五金工具收纳_镂空1 (Autodesk Fusion 360 design; units mm, degrees)
part number: 2026-02-27-19-53-02-708
Autodesk Fusion 360 part; units mm, degrees
(part 1 of 9)
sketch "草图1" plane through (0, 0, 0) normal (0, 0, 1) x (1, 0, 0)
  line L0 (-120, 120) -> (120, 120)
  line L1 (120, 120) -> (120, -120)
  line L2 (120, -120) -> (-120, -120)
  line L3 (-120, -120) -> (-120, 120)
  line L4 (-120, 120) -> (120, -120) construction
  line L5 (120, 120) -> (-120, -120) construction
  line L6 (-116, -116) -> (-116, 116)
  line L7 (-116, 116) -> (116, 116)
  line L8 (116, 116) -> (116, -116)
  line L9 (116, -116) -> (-116, -116)
  line L10 (-116, 116) -> (4, 116)
  line L11 (4, 116) -> (4, -4)
  line L12 (4, -4) -> (-116, -4)
  line L13 (-116, -4) -> (-116, 116)
  line L14 (7, 116) -> (7, -7)
  line L15 (7, -7) -> (-116, -7)
  line L16 (-91.3834, 29.143) -> (-25.513, 29.143) construction
  line L17 (-25.513, 29.143) -> (-25.513, 88.3753) construction
  line L18 (-25.513, 88.3753) -> (-91.3834, 88.3753) construction
  line L19 (-91.3834, 88.3753) -> (-91.3834, 29.143) construction
  line L20 (7, 80) -> (72, 80)
  line L21 (72, 80) -> (72, 116)
  line L22 (7, 83) -> (69, 83)
  line L23 (69, 83) -> (69, 116)
  line L24 (25.1429, 88.9882) -> (53.1683, 88.9882) construction
  line L25 (53.1683, 88.9882) -> (53.1683, 99.6185) construction
  line L26 (53.1683, 99.6185) -> (25.1429, 99.6185) construction
  line L27 (25.1429, 99.6185) -> (25.1429, 88.9882) construction
  line L28 (67, 80) -> (67, 57)
  line L29 (67, 57) -> (7, 57)
  line L30 (17, 80) -> (57, 80)
  line L31 (57, 80) -> (57, 60)
  line L32 (57, 60) -> (17, 60)
  line L33 (17, 60) -> (17, 80)
  line L34 (26, 65.6005) -> (48.0911, 65.6005) construction
  line L35 (48.0911, 65.6005) -> (48.0911, 73) construction
  line L36 (48.0911, 73) -> (26, 73) construction
  line L37 (26, 73) -> (26, 65.6005) construction
  line L38 (-116, -7) -> (-41, -7)
  line L39 (-41, -7) -> (-41, -82)
  line L40 (-41, -82) -> (-116, -82)
  line L41 (-116, -82) -> (-116, -7)
  line L42 (-38, -7) -> (-38, -85)
  line L43 (-38, -85) -> (-116, -85)
  line L44 (-99.1433, -54.3081) -> (-63.0106, -54.3081) construction
  line L45 (-63.0106, -54.3081) -> (-63.0106, -32.999) construction
  line L46 (-63.0106, -32.999) -> (-99.1433, -32.999) construction
  line L47 (-99.1433, -32.999) -> (-99.1433, -54.3081) construction
  line L48 (7, 57) -> (67, 57)
  line L49 (67, 57) -> (67, 37)
  line L50 (67, 37) -> (7, 37)
  line L51 (7, 37) -> (7, 57)
  line L52 (64, 57) -> (64, 40)
  line L53 (64, 40) -> (7, 40)
  line L54 (25.5114, 42.6447) -> (56.3611, 42.6447) construction
  line L55 (56.3611, 42.6447) -> (56.3611, 51.3132) construction
  line L56 (56.3611, 51.3132) -> (25.5114, 51.3132) construction
  line L57 (25.5114, 51.3132) -> (25.5114, 42.6447) construction
  line L58 (72, 103) -> (116, 103)
  line L59 (72, 87) -> (116, 87)
  line L60 (72, 100) -> (116, 100)
  line L61 (72, 84) -> (116, 84)
  line L62 (67, 71) -> (116, 71)
  line L63 (67, 40) -> (116, 40)
  line L64 (67, 68) -> (116, 68)
  line L65 (67, 37) -> (116, 37)
  line L66 (76.846, 102.1326) -> (102.0197, 102.0197) construction
  line L67 (102.0197, 102.0197) -> (102.0756, 114.498) construction
  line L68 (102.0756, 114.498) -> (76.902, 114.6109) construction
  line L69 (76.902, 114.6109) -> (76.846, 102.1326) construction
  line L70 (84.3585, 90.542) -> (111.7961, 90.6188) construction
  line L71 (111.7961, 90.6188) -> (111.7764, 97.6581) construction
  line L72 (111.7764, 97.6581) -> (84.3388, 97.5814) construction
  line L73 (84.3388, 97.5814) -> (84.3585, 90.542) construction
  line L74 (94.1738, 75) -> (110, 75) construction
  line L75 (110, 75) -> (110, 79.4268) construction
  line L76 (110, 79.4268) -> (94.1738, 79.4268) construction
  line L77 (94.1738, 79.4268) -> (94.1738, 75) construction
  line L78 (80, 47.31) -> (108.2637, 47.31) construction
  line L79 (108.2637, 47.31) -> (108.2637, 60) construction
  line L80 (108.2637, 60) -> (80, 60) construction
  line L81 (80, 60) -> (80, 47.31) construction
  line L82 (-85, -85) -> (-85, -116)
  line L83 (-54, -85) -> (-54, -116)
  line L84 (-38, -85) -> (-5, -85)
  line L85 (-5, -85) -> (-5, -116)
  line L86 (-23, -85) -> (-23, -116)
  line L87 (-116, -85) -> (-85, -116) construction
  line L88 (-54, -85) -> (-85, -116) construction
  line L89 (-85, -85) -> (-54, -116) construction
  line L90 (-54, -85) -> (-23, -116) construction
  line L91 (-23, -116) -> (-5, -85) construction
  line L92 (-23, -85) -> (-5, -116) construction
  line L93 (-23, -85) -> (-54, -116) construction
  circle A0 centre (-100.5, -100.5) radius 3.65
  circle A1 centre (-69.5, -100.5) radius 3.65
  circle A2 centre (-38.5, -100.5) radius 2.25
  circle A3 centre (-14, -100.5) radius 2.5
  line L94 (72, 6) -> (7, 6)
  line L95 (72, 12) -> (72, 6)
  line L96 (26.8319, 6.972) -> (48.9756, 6.972) construction
  line L97 (48.9756, 6.972) -> (48.9756, 11.0156) construction
  line L98 (48.9756, 11.0156) -> (26.8319, 11.0156) construction
  line L99 (26.8319, 11.0156) -> (26.8319, 6.972) construction
  line L100 (40.1808, 17.1326) -> (43.385, 17.1326) construction
  line L101 (43.385, 17.1326) -> (43.385, 35.2897) construction
  line L102 (43.385, 35.2897) -> (40.1808, 35.2897) construction
  line L103 (40.1808, 35.2897) -> (40.1808, 17.1326) construction
  line L104 (18.6537, 18.964) -> (25.5317, 18.964) construction
  line L105 (25.5317, 18.964) -> (25.5317, 32.3581) construction
  line L106 (25.5317, 32.3581) -> (18.6537, 32.3581) construction
  line L107 (18.6537, 32.3581) -> (18.6537, 18.964) construction
  line L108 (35, 37) -> (35, 12)
  line L109 (35, 12) -> (7, 12)
  line L110 (32, 15) -> (7, 15)
  line L111 (32, 37) -> (32, 15)
  line L112 (35, 15) -> (67, 15)
  line L113 (67, 15) -> (67, 37)
  line L114 (35, 12) -> (70, 12)
  line L115 (70, 12) -> (70, 37)
  line L116 (70, 30) -> (116, 30)
  line L117 (70, 27) -> (116, 27)
  line L118 (79.0707, 32.0224) -> (93.9955, 32.0224) construction
  line L119 (93.9955, 32.0224) -> (93.9955, 35.3609) construction
  line L120 (93.9955, 35.3609) -> (79.0707, 35.3609) construction
  line L121 (79.0707, 35.3609) -> (79.0707, 32.0224) construction
  line L122 (7, -7) -> (116, -7)
  line L123 (116, -7) -> (116, -116)
  line L124 (116, -116) -> (7, -116)
  line L125 (7, -116) -> (7, -7)
  line L126 (7, 116) -> (7, 120)
  line L127 (-116, -7) -> (-121.1752, -7)
  line L128 (72, 116) -> (72, 120)
  line L129 (116, 100) -> (120, 100)
  line L130 (116, 84) -> (120, 84)
  line L131 (69, 116) -> (69, 120)
  line L132 (72, 100) -> (69, 100)
  line L133 (72, 84) -> (69, 84)
  line L134 (-38, -7) -> (-38, -4)
  line L135 (-116, -85) -> (-120, -85)
  line L136 (-116, -4) -> (-120, -4)
  line L137 (86.5, 23) -> (86.5, -4)
  line L138 (74.7536, 23) -> (74.7536, 3)
  line L139 (84, -4.0797) -> (84, 23)
  line L140 (113.5, -4) -> (113.5, 23)
  line L141 (86.5, -4) -> (113.5, -4)
  line L142 (113.5, 23) -> (86.5, 23)
  line L143 (84, 23) -> (74.7536, 23)
  line L144 (7, -4.0797) -> (84, -4.0797)
  line L145 (74.7536, 3) -> (7, 3)
  line L146 (7, 3) -> (7, -4.0797)
  line L147 (4.0918, -82) -> (-38, -82)
  line L148 (-38, -7) -> (4, -7)
  line L149 (-38, -27) -> (-38, -7)
  line L150 (-38, -50) -> (-38, -30)
  line L151 (-38, -30) -> (4, -30)
  line L152 (-38, -82) -> (-38, -54.2912)
  line L153 (4, -27) -> (-38, -27)
  line L154 (4, -50) -> (-38, -50)
  line L155 (-38, -54.2912) -> (4.0918, -54.2912)
  line L156 (4.0918, -54.2912) -> (4.0918, -82)
  line L157 (4, -30) -> (4, -50)
  line L158 (4, -7) -> (4, -27)
  line L159 (72, 12) -> (70, 12)
  line L160 (84, -4.0797) -> (116, -4.0797)
  line L161 (4, -7) -> (4, -120)
  line L162 (116, -4.0797) -> (120, -4.0797)
  circle A4 centre (-38.5, -100.5) radius 5.25
  circle A5 centre (-69.5, -100.5) radius 6.65
  circle A6 centre (-100.5, -100.5) radius 6.65
  circle A7 centre (-14, -100.5) radius 5.5
  point P0 (66.165, 12.6159)
  point P1 (18.6537, 18.964)
  point P2 (18.6537, 32.3581)
  point P3 (25.5317, 18.964)
  point P4 (25.5317, 32.3581)
  point P5 (-108.25, 88.6913)
  dimension "d22" = 240
  dimension "d23" = 240
  dimension "d24" = 4
  dimension "d25" = 120
  dimension "d26" = 120
  dimension "d28" = 10
  dimension "d45" = 65
  dimension "d46" = 36
  dimension "d47" = -3
  dimension "d48" = 5
  dimension "d50" = 44
  dimension "d51" = 60
  dimension "d52" = 23
  dimension "d54" = 40
  dimension "d55" = 20
  dimension "d56" = 10
  dimension "d57" = 5
  dimension "d60" = 75
  dimension "d61" = 75
  dimension "d62" = -3
  dimension "d63" = 5
  dimension "d65" = 60
  dimension "d66" = 20
  dimension "d67" = 3
  dimension "d68" = 5
  dimension "d70" = 13
  dimension "d76" = 3
  dimension "d77" = 3
  dimension "d80" = 13
  dimension "d81" = 3
  dimension "d82" = 3
  dimension "d84" = 5
  dimension "d86" = 5
  dimension "d88" = 5
  dimension "d90" = 5
  dimension "d92" = 13
  dimension "d93" = 60
  dimension "d100" = 31
  dimension "d101" = 31
  dimension "d102" = 31
  dimension "d103" = 31
  dimension "d104" = 18
  dimension "d105" = 7.3
  dimension "d106" = 7.3
  dimension "d107" = 4.5
  dimension "d108" = 5
  dimension "d119" = 5
  dimension "d122" = 5
  dimension "d125" = 5
  dimension "d127" = -3
  dimension "d128" = 25
  dimension "d129" = 22
  dimension "d131" = 32
  dimension "d132" = 22
  dimension "d133" = 3
  dimension "d134" = 7
  dimension "d135" = 3
  dimension "d136" = 5
  dimension "d138" = 109
  dimension "d139" = 109
  dimension "d144" = 65
  dimension "d145" = 6
  dimension "d255" = 27
  dimension "d256" = 27
  dimension "d257" = 42
  dimension "d258" = 20
  dimension "d259" = 42
  dimension "d260" = 20
  dimension "d261" = 3
  dimension "d263" = 2.5
  dimension "d264" = 2.5
  dimension "d265" = 4
  dimension "d275" = 3
  dimension "d276" = 3
  dimension "d277" = 3
  dimension "d280" = 3
  constraint horizontal L0
  constraint perpendicular L0 L1
  constraint parallel L0 L2
  constraint parallel L1 L3
  constraint coincident L4 origin
  constraint coincident L5 origin
  constraint horizontal L10
  constraint vertical L11
  constraint horizontal L12
  constraint vertical L13
  constraint coincident L7 L14.start
  constraint coincident L6 L15.end
  constraint coincident L14 L20.start
  constraint perpendicular L14 L20
  constraint coincident L7 L21.end
  constraint perpendicular L7 L21
  constraint coincident L20 L28.start
  constraint perpendicular L20 L28
  constraint coincident L14 L29.end
  constraint perpendicular L14 L29
  constraint horizontal L30
  constraint vertical L31
  constraint horizontal L32
  constraint vertical L33
  constraint coincident L20 L30.start
  constraint horizontal L38
  constraint vertical L39
  constraint horizontal L40
  constraint vertical L41
  constraint horizontal L48
  constraint vertical L49
  constraint horizontal L50
  constraint vertical L51
  constraint coincident L21 L58.start
  constraint perpendicular L8 L58
  constraint coincident L8 L58.end
  constraint coincident L28 L62.start
  constraint coincident L8 L62.end
  constraint perpendicular L8 L62
  constraint coincident L49 L63.start
  constraint coincident L8 L63.end
  constraint perpendicular L8 L63
  constraint coincident L5
  constraint coincident L50 L49.end
  constraint coincident L43 L82.start
  constraint coincident L9 L82.end
  constraint perpendicular L9 L82
  constraint coincident L43 L83.start
  constraint coincident L9 L83.end
  constraint perpendicular L9 L83
  constraint perpendicular L42 L84
  constraint coincident L9 L85.end
  constraint perpendicular L9 L85
  constraint coincident L84 L86.start
  constraint coincident L9 L86.end
  constraint perpendicular L9 L86
  constraint perpendicular L5 L87
  constraint midpoint L87 A0.centre
  constraint midpoint L89 A1.centre
  constraint midpoint L93 A2.centre
  constraint midpoint L91 A3.centre
  constraint coincident L50 L111.start
  constraint coincident L14 L110.end
  constraint perpendicular L110 L111
  constraint coincident L108 L112.start
  constraint perpendicular L101 L112
  constraint perpendicular L50 L113
  constraint coincident L115 L116.start
  constraint coincident L8 L116.end
  constraint perpendicular L8 L116
  constraint horizontal L122
  constraint vertical L123
  constraint horizontal L124
  constraint vertical L125
  constraint perpendicular L94 L95
  constraint coincident L0 L126.end
  constraint perpendicular L0 L126
  constraint perpendicular L3 L127
  constraint coincident L0 L128.end
  constraint perpendicular L0 L128
  constraint coincident L1 L129.end
  constraint perpendicular L1 L129
  constraint coincident L1 L130.end
  constraint perpendicular L1 L130
  constraint coincident L0 L131.end
  constraint perpendicular L0 L131
  constraint coincident L23 L132.end
  constraint perpendicular L23 L132
  constraint coincident L23 L133.end
  constraint perpendicular L23 L133
  constraint coincident L12 L134.end
  constraint perpendicular L12 L134
  constraint coincident L3 L135.end
  constraint perpendicular L3 L135
  constraint coincident L3 L136.end
  constraint perpendicular L3 L136
  constraint horizontal L141
  constraint vertical L140
  constraint horizontal L142
  constraint vertical L137
  constraint vertical L146
  constraint perpendicular L144 L146
  constraint perpendicular L139 L144
  constraint perpendicular L139 L143
  constraint perpendicular L138 L143
  constraint horizontal L145
  constraint horizontal L153
  constraint vertical L149
  constraint horizontal L151
  constraint vertical L157
  constraint horizontal L154
  constraint vertical L150
  constraint horizontal L155
  constraint vertical L156
  constraint horizontal L147
  constraint vertical L152
  constraint collinear L149 L150
  constraint collinear L150 L152
  constraint collinear L142 L143
  constraint collinear L14 L146
  constraint coincident L8 L160.end
  constraint perpendicular L8 L160
  constraint coincident L2 L161.end
  constraint perpendicular L2 L161
  constraint coincident L1 L162.end
  constraint perpendicular L1 L162
  measures "d22" distance of L1.end L2.end
  measures "d23" distance of L0.end L1.end
  measures "d25" distance of L6.end L10.end
  measures "d26" distance of L6.end L12.end
  measures "d45" distance of L14 L21
  measures "d46" distance of L7 L20
  measures "d50" distance of L8 L21
  measures "d51" distance of L14 L28
  measures "d52" distance of L20 L29
  measures "d54" distance of L30.start L30.end
  measures "d55" distance of L30.start L32.end
  measures "d56" distance of L14 L33
  measures "d60" distance of L15.end L38.end
  measures "d61" distance of L15.end L40.end
  measures "d65" distance of L29.end L28.end
  measures "d66" distance of L29.end L50.end
  measures "d70" distance of L7 L58
  measures "d80" distance of L61 L62
  measures "d92" distance of L59 L60
  measures "d93" distance of L14 L28
  measures "d100" distance of L9 L43
  measures "d101" distance of L6 L82
  measures "d102" distance of L82 L83
  measures "d103" distance of L83 L86
  measures "d104" distance of L85 L86
  measures "d105" diameter of A0
  measures "d106" diameter of A1
  measures "d107" diameter of A2
  measures "d108" diameter of A3
  measures "d128" distance of L14 L111
  measures "d129" distance of L50 L110
  measures "d131" distance of L112.start L112.end
  measures "d132" distance of L50 L112
  measures "d134" distance of L65 L116
  measures "d138" distance of L9 L122
  measures "d139" distance of L8 L125
  measures "d144" distance of L14 L95
  measures "d145" distance of L94 L114
  measures "d255" distance of L137.end L140.start
  measures "d256" distance of L137.end L137.start
  measures "d257" distance of L42.start L148.end
  measures "d258" distance of L42.start L149.start
  measures "d259" distance of L151.end L150.end
  measures "d260" distance of L150.end L150.start
  measures "d261" distance of L151 L153
  measures "d263" distance of L8 L140
  measures "d264" distance of L137 L139
  measures "d265" distance of L117 L142
sketch "草图2" plane through (0, 0, 0) normal (0, 0, 1) x (1, 0, 0)
  line L0 (-120, 120) -> (120, 120)
  line L1 (120, 120) -> (120, -120)
  line L2 (120, -120) -> (-120, -120)
  line L3 (-120, -120) -> (-120, 120)
  circle A0 centre (-14, -100.5) radius 2.5
  circle A1 centre (-38.5, -100.5) radius 2.25
  circle A2 centre (-69.5, -100.5) radius 3.65
  circle A3 centre (-100.5, -100.5) radius 3.65
  line L4 (3.9913, -3.998) -> (-116.0052, -3.998)
  line L5 (3.9913, 116.0345) -> (3.9913, -3.998)
  line L6 (7.0361, -7.055) -> (116, -7.055)
  line L7 (7.0361, -116.055) -> (7.0361, -7.055)
  line L8 (-116.0087, 116.002) -> (3.9913, 116.0345)
  line L9 (-116.0052, -3.998) -> (-116.0087, 116.002)
  line L10 (116, -7.055) -> (116, -116.055)
  line L11 (116, -116.055) -> (7.0361, -116.055)
  line L12 (-41, -7) -> (-41, -82)
  line L13 (-41, -82) -> (-116, -82)
  line L14 (-116, -116) -> (-116, 116.0345)
  line L15 (-41, -7) -> (-116, -7)
  line L16 (32, 37) -> (32, 15)
  line L17 (32, 15) -> (7, 15)
  line L18 (35, 15) -> (67, 15)
  line L19 (67, 15) -> (67, 37)
  line L20 (35, 37) -> (35, 15)
  line L21 (72, 6) -> (7, 6)
  line L22 (72, 12) -> (72, 6)
  line L23 (35, 12) -> (70, 12)
  line L24 (35, 12) -> (7, 12)
  line L25 (70, 30) -> (116, 30)
  line L26 (70, 30) -> (70, 37)
  line L27 (67, 40) -> (116, 40)
  line L28 (67, 57) -> (67, 40)
  line L29 (67, 68.0345) -> (116, 68.0345)
  line L30 (64, 57) -> (64, 39.9995)
  line L31 (64, 39.9995) -> (7, 39.9995)
  line L32 (57, 80.0345) -> (57, 60.0345)
  line L33 (57, 60.0345) -> (17, 60.0345)
  line L34 (17, 60.0345) -> (17, 80.0345)
  line L35 (7, 83.0345) -> (69, 83.0345)
  line L36 (69, 83.0345) -> (69, 116.005)
  line L37 (17, 80.0345) -> (57, 80.0345)
  line L38 (72, 84.0345) -> (116, 84.0345)
  line L39 (67, 71.0345) -> (116, 71.0345)
  line L40 (72, 87.0345) -> (116, 87.0345)
  line L41 (72, 103.0345) -> (116, 103.0345)
  line L42 (72, 100.0345) -> (116, 100.0345)
  line L43 (3.5986, -3.998) -> (3.9913, -3.998)
  line L44 (7, 12) -> (7, 6)
  line L45 (7, 37) -> (7, 15)
  line L46 (32, 37) -> (7, 37)
  line L47 (67, 37) -> (35, 37)
  line L48 (70, 37) -> (116, 37)
  line L49 (72, 12) -> (70, 12)
  line L50 (67, 68.0345) -> (67, 57)
  line L51 (67, 80.0345) -> (67, 71.0345)
  line L52 (116, 100.0345) -> (116, 87.0345)
  line L53 (116, 116.0403) -> (116, 103.0345)
  line L54 (72, 103.0345) -> (72, 116.0345)
  line L55 (72, 80.0368) -> (72, 84.0345)
  line L56 (72, 87.0345) -> (72, 100.0345)
  line L57 (17, 80.0345) -> (57, 80.0345)
  line L58 (67, 80.0345) -> (72, 80.0368)
  line L59 (-116, 116.0345) -> (3.9913, 116.0345)
  line L60 (7, 116.0345) -> (69, 116.005)
  line L61 (72, 116.0345) -> (116, 116.0403)
  line L62 (7, 116.0345) -> (7, 83.0345)
  line L63 (7, 57) -> (7, 39.9995)
  line L64 (116, 84.0345) -> (116, 71.0345)
  line L65 (116, -7.055) -> (116, -116)
  line L66 (116, 68.0345) -> (116, 40)
  line L67 (116, 37) -> (116, 30)
  line L68 (7, 57) -> (64, 57)
  line L69 (-38, -7) -> (4, -7)
  line L70 (4, -7) -> (4, -27)
  line L71 (4, -27) -> (-38, -27)
  line L72 (-38, -27) -> (-38, -7)
  line L73 (4, -30) -> (4, -50)
  line L74 (-38, -50) -> (-38, -30)
  line L75 (4, -50) -> (-38, -50)
  line L76 (-38, -30) -> (4, -30)
  line L77 (-38, -54.2912) -> (4.0918, -54.2912)
  line L78 (4.0918, -54.2912) -> (4.0918, -82)
  line L79 (4.0918, -82) -> (-38, -82)
  line L80 (-38, -82) -> (-38, -54.2912)
  line L81 (113.5, 23) -> (86.5, 23)
  line L82 (74.7536, 23) -> (74.7536, 3)
  line L83 (113.5, -4) -> (113.5, 23)
  line L84 (84, -4.0797) -> (84, 23)
  line L85 (86.5, -4) -> (113.5, -4)
  line L86 (86.5, 23) -> (86.5, -4)
  line L87 (84, 23) -> (74.7536, 23)
  line L88 (74.7536, 3) -> (7, 3)
  line L89 (7, -4.0797) -> (84, -4.0797)
  line L90 (7, 3) -> (7, -4.0797)
  line L91 (7, 116) -> (7, 83.0345)
  line L92 (7, 57) -> (7, 39.9995)
  line L93 (7, 37) -> (7, 6)
  dimension "d176" = 7.3
  dimension "d177" = 7.3
  dimension "d178" = 4.5
  dimension "d179" = 5
  dimension "d180" = 120
  dimension "d181" = 120
  dimension "d186" = 3
  dimension "d187" = 3
  dimension "d188" = 3
  dimension "d193" = 65
  dimension "d194" = 36
  dimension "d197" = 40
  dimension "d198" = 20
  dimension "d199" = 10
  dimension "d200" = 75
  dimension "d201" = 75
  dimension "d202" = 13
  dimension "d203" = 13
  dimension "d204" = 13
  dimension "d206" = 25
  dimension "d208" = 32
  dimension "d212" = 65
  dimension "d213" = 6
  dimension "d215" = 3
  dimension "d227" = 42
  dimension "d228" = 20
  dimension "d230" = 42
  dimension "d231" = 20
  dimension "d232" = 3.002
  dimension "d233" = 3
  dimension "d236" = 3
  dimension "d266" = 27
  dimension "d267" = 27
  dimension "d268" = 2.5
  constraint horizontal L0
  constraint vertical L1
  constraint horizontal L2
  constraint vertical L3
  constraint vertical L5
  constraint horizontal L4
  constraint horizontal L6
  constraint vertical L7
  constraint coincident L60.start L59
  constraint coincident L15.end L14
  constraint perpendicular L57 L63
  constraint coincident L54.end L59
  constraint perpendicular L55 L59
  constraint coincident L51.start L57
  constraint horizontal L37
  constraint vertical L32
  constraint horizontal L33
  constraint vertical L34
  constraint vertical L12
  constraint horizontal L13
  constraint vertical L28
  constraint coincident L17.end L63
  constraint perpendicular L16 L17
  constraint perpendicular L21 L22
  constraint horizontal L46
  constraint horizontal L47
  constraint coincident L26 L48.start
  constraint perpendicular L50 L57
  constraint perpendicular L51 L57
  constraint perpendicular L41 L53
  constraint perpendicular L54 L59
  constraint collinear L62 L63
  constraint coincident L39 L64.end
  constraint collinear L64 L66
  constraint coincident L25 L67.end
  constraint collinear L65 L67
  constraint coincident L27 L66.end
  constraint collinear L66 L67
  constraint horizontal L68
  constraint horizontal L71
  constraint vertical L72
  constraint horizontal L76
  constraint vertical L73
  constraint horizontal L75
  constraint vertical L74
  constraint horizontal L77
  constraint vertical L78
  constraint horizontal L79
  constraint vertical L80
  constraint collinear L72 L74
  constraint collinear L74 L80
  constraint collinear L13 L79
  constraint horizontal L85
  constraint vertical L83
  constraint horizontal L81
  constraint vertical L86
  constraint perpendicular L84 L89
  constraint perpendicular L84 L87
  constraint perpendicular L82 L87
  constraint horizontal L88
  constraint collinear L81 L87
  constraint collinear L90 L93
  constraint collinear L91 L92
  constraint collinear L92 L93
  measures "d176" diameter of A3
  measures "d177" diameter of A2
  measures "d178" diameter of A1
  measures "d179" diameter of A0
  measures "d180" distance of L5.start L8.start
  measures "d181" distance of L4.end L8.start
  measures "d193" distance of L55 L62
  measures "d194" distance of L57 L59
  measures "d197" distance of L34.end L32.start
  measures "d198" distance of L34.end L33.end
  measures "d199" distance of L34 L63
  measures "d200" distance of L15.end L12.start
  measures "d201" distance of L15.end L13.end
  measures "d202" distance of L41 L59
  measures "d203" distance of L38 L39
  measures "d204" distance of L40 L42
  measures "d206" distance of L16 L63
  measures "d208" distance of L18.start L18.end
  measures "d212" distance of L22 L63
  measures "d213" distance of L21 L23
  measures "d215" distance of L27 L47
  measures "d227" distance of L69.start L69.end
  measures "d228" distance of L69.start L71.end
  measures "d230" distance of L74.end L73.start
  measures "d231" distance of L74.end L74.start
  measures "d232" distance of L4 L69
  measures "d233" distance of L71 L76
  measures "d236" distance of L12 L72
  measures "d266" distance of L83.start L85.start
  measures "d267" distance of L81.end L85.start
  measures "d268" distance of L84 L86
sketch "草图3" plane through (0, 0, 0) normal (0, 0, 1) x (1, 0, 0)
  line L0 (-120, 120) -> (120, 120)
  line L1 (-120, -120) -> (-120, 120)
  line L2 (120, 120) -> (120, -120)
  line L3 (120, -120) -> (-120, -120)
  point P0 (116, 40)
  constraint horizontal L0
  constraint vertical L2
  constraint horizontal L3
  constraint vertical L1
extrude "拉伸2" add sketch "草图3" against normal blind 5 makes body 1
extrude "拉伸3" add sketch "草图2" along normal blind 65 bodies 1
extrude "拉伸4" add sketch "草图1" along normal blind 160 contours L0 L3 L6 L7 L10 L13 L126 L136 | L3 L6 L127 L136 | L7 L11 L12 L14 L15 L51 L134 L146 L148 | L6 L12 L15 L38 L134 bodies 1
extrude "拉伸5" add sketch "草图1" along normal blind 90 contours L0 L7 L126 L131 | L0 L7 L128 L131 | L7 L21 L23 L132 | L14 L20 L21 L22 L23 L30 L133 | L21 L23 L132 L133 | L14 L20 L28 L29 L31 L32 L33 L48 bodies 1
extrude "拉伸6" add sketch "草图1" along normal blind 140 contours L0 L1 L7 L8 L128 L129 | L8 L21 L58 L60 bodies 1
extrude "拉伸7" add sketch "草图1" along normal blind 140 contours L0 L7 L128 L131 | L7 L21 L23 L132 bodies 1
extrude "拉伸8" add sketch "草图1" along normal blind 80 separate body contours L1 L8 L129 L130 | L8 L21 L59 L61 makes body 2
extrude "拉伸9" add sketch "草图1" along normal blind 140 separate body contours L3 L6 L127 L136 | L3 L6 L41 L127 L135 | L6 L12 L15 L38 L134 | L6 L15 L39 L40 L42 L43 L149 L150 L152 makes body 3
extrude "拉伸10" add sketch "草图1" along normal blind 120 separate body contours L1 L2 L8 L9 L123 L124 L161 L162 | L9 L15 L125 L147 L155 L156 L157 L158 L161 | L8 L14 L122 L144 L160 makes body 4
extrude "拉伸11" cut sketch "草图1" along normal blind 70 contours L9 L84 L85 L86 | A7 bodies 1
extrude "拉伸12" add sketch "草图1" along normal blind 40 separate body contours L9 L84 L85 L86 | A7 makes body 5
extrude "拉伸13" cut sketch "草图1" along normal blind 60 contours L6 L9 L43 L82 | L9 L43 L82 L83 | L9 L43 L83 L84 L86 bodies 1
extrude "拉伸14" cut sketch "草图1" along normal blind 30 contours L9 L84 L85 L86 bodies 5
sketch "草图20" plane through (4, 0, 0) normal (-1, 0, 0) x (0, -1, 0)
  line L0 (-116, 65) -> (4, 65)
  line L1 (4, 65) -> (4, 160)
  line L2 (4, 160) -> (-116, 160)
  line L3 (-116, 160) -> (-116, 65)
  line L4 (-109, 77) -> (-113.3301, 74.5)
  line L5 (-113.3301, 74.5) -> (-113.3301, 69.5)
  line L6 (-113.3301, 69.5) -> (-109, 67)
  line L7 (-109, 67) -> (-104.6699, 69.5)
  line L8 (-104.6699, 69.5) -> (-104.6699, 74.5)
  line L9 (-104.6699, 74.5) -> (-109, 77)
  line L10 (-98.8397, 77) -> (-103.1699, 74.5)
  line L11 (-103.1699, 74.5) -> (-103.1699, 69.5)
  line L12 (-103.1699, 69.5) -> (-98.8397, 67)
  line L13 (-98.8397, 67) -> (-94.5096, 69.5)
  line L14 (-94.5096, 69.5) -> (-94.5096, 74.5)
  line L15 (-94.5096, 74.5) -> (-98.8397, 77)
  line L16 (-88.6795, 77) -> (-93.0096, 74.5)
  line L17 (-93.0096, 74.5) -> (-93.0096, 69.5)
  line L18 (-93.0096, 69.5) -> (-88.6795, 67)
  line L19 (-88.6795, 67) -> (-84.3494, 69.5)
  line L20 (-84.3494, 69.5) -> (-84.3494, 74.5)
  line L21 (-84.3494, 74.5) -> (-88.6795, 77)
  line L22 (-78.5192, 77) -> (-82.8494, 74.5)
  line L23 (-82.8494, 74.5) -> (-82.8494, 69.5)
  line L24 (-82.8494, 69.5) -> (-78.5192, 67)
  line L25 (-78.5192, 67) -> (-74.1891, 69.5)
  line L26 (-74.1891, 69.5) -> (-74.1891, 74.5)
  line L27 (-74.1891, 74.5) -> (-78.5192, 77)
  line L28 (-68.359, 77) -> (-72.6891, 74.5)
  line L29 (-72.6891, 74.5) -> (-72.6891, 69.5)
  line L30 (-72.6891, 69.5) -> (-68.359, 67)
  line L31 (-68.359, 67) -> (-64.0289, 69.5)
  line L32 (-64.0289, 69.5) -> (-64.0289, 74.5)
  line L33 (-64.0289, 74.5) -> (-68.359, 77)
  line L34 (-58.1987, 77) -> (-62.5289, 74.5)
  line L35 (-62.5289, 74.5) -> (-62.5289, 69.5)
  line L36 (-62.5289, 69.5) -> (-58.1987, 67)
  line L37 (-58.1987, 67) -> (-53.8686, 69.5)
  line L38 (-53.8686, 69.5) -> (-53.8686, 74.5)
  line L39 (-53.8686, 74.5) -> (-58.1987, 77)
  line L40 (-48.0385, 77) -> (-52.3686, 74.5)
  line L41 (-52.3686, 74.5) -> (-52.3686, 69.5)
  line L42 (-52.3686, 69.5) -> (-48.0385, 67)
  line L43 (-48.0385, 67) -> (-43.7084, 69.5)
  line L44 (-43.7084, 69.5) -> (-43.7084, 74.5)
  line L45 (-43.7084, 74.5) -> (-48.0385, 77)
  line L46 (-37.8782, 77) -> (-42.2084, 74.5)
  line L47 (-42.2084, 74.5) -> (-42.2084, 69.5)
  line L48 (-42.2084, 69.5) -> (-37.8782, 67)
  line L49 (-37.8782, 67) -> (-33.5481, 69.5)
  line L50 (-33.5481, 69.5) -> (-33.5481, 74.5)
  line L51 (-33.5481, 74.5) -> (-37.8782, 77)
  line L52 (-27.718, 77) -> (-32.0481, 74.5)
  line L53 (-32.0481, 74.5) -> (-32.0481, 69.5)
  line L54 (-32.0481, 69.5) -> (-27.718, 67)
  line L55 (-27.718, 67) -> (-23.3878, 69.5)
  line L56 (-23.3878, 69.5) -> (-23.3878, 74.5)
  line L57 (-23.3878, 74.5) -> (-27.718, 77)
  line L58 (-17.5577, 77) -> (-21.8878, 74.5)
  line L59 (-21.8878, 74.5) -> (-21.8878, 69.5)
  line L60 (-21.8878, 69.5) -> (-17.5577, 67)
  line L61 (-17.5577, 67) -> (-13.2276, 69.5)
  line L62 (-13.2276, 69.5) -> (-13.2276, 74.5)
  line L63 (-13.2276, 74.5) -> (-17.5577, 77)
  line L64 (-7.3975, 77) -> (-11.7276, 74.5)
  line L65 (-11.7276, 74.5) -> (-11.7276, 69.5)
  line L66 (-11.7276, 69.5) -> (-7.3975, 67)
  line L67 (-7.3975, 67) -> (-3.0673, 69.5)
  line L68 (-3.0673, 69.5) -> (-3.0673, 74.5)
  line L69 (-3.0673, 74.5) -> (-7.3975, 77)
  line L70 (-103.9199, 85.799) -> (-108.25, 83.299)
  line L71 (-108.25, 83.299) -> (-108.25, 78.299)
  line L72 (-108.25, 78.299) -> (-103.9199, 75.799)
  line L73 (-103.9199, 75.799) -> (-99.5897, 78.299)
  line L74 (-99.5897, 78.299) -> (-99.5897, 83.299)
  line L75 (-99.5897, 83.299) -> (-103.9199, 85.799)
  line L76 (-93.7596, 85.799) -> (-98.0897, 83.299)
  line L77 (-98.0897, 83.299) -> (-98.0897, 78.299)
  line L78 (-98.0897, 78.299) -> (-93.7596, 75.799)
  line L79 (-93.7596, 75.799) -> (-89.4295, 78.299)
  line L80 (-89.4295, 78.299) -> (-89.4295, 83.299)
  line L81 (-89.4295, 83.299) -> (-93.7596, 85.799)
  line L82 (-83.5994, 85.799) -> (-87.9295, 83.299)
  line L83 (-87.9295, 83.299) -> (-87.9295, 78.299)
  line L84 (-87.9295, 78.299) -> (-83.5994, 75.799)
  line L85 (-83.5994, 75.799) -> (-79.2692, 78.299)
  line L86 (-79.2692, 78.299) -> (-79.2692, 83.299)
  line L87 (-79.2692, 83.299) -> (-83.5994, 85.799)
  line L88 (-73.4391, 85.799) -> (-77.7692, 83.299)
  line L89 (-77.7692, 83.299) -> (-77.7692, 78.299)
  line L90 (-77.7692, 78.299) -> (-73.4391, 75.799)
  line L91 (-73.4391, 75.799) -> (-69.109, 78.299)
  line L92 (-69.109, 78.299) -> (-69.109, 83.299)
  line L93 (-69.109, 83.299) -> (-73.4391, 85.799)
  line L94 (-63.2789, 85.799) -> (-67.609, 83.299)
  line L95 (-67.609, 83.299) -> (-67.609, 78.299)
  line L96 (-67.609, 78.299) -> (-63.2789, 75.799)
  line L97 (-63.2789, 75.799) -> (-58.9487, 78.299)
  line L98 (-58.9487, 78.299) -> (-58.9487, 83.299)
  line L99 (-58.9487, 83.299) -> (-63.2789, 85.799)
  line L100 (-53.1186, 85.799) -> (-57.4487, 83.299)
  line L101 (-57.4487, 83.299) -> (-57.4487, 78.299)
  line L102 (-57.4487, 78.299) -> (-53.1186, 75.799)
  line L103 (-53.1186, 75.799) -> (-48.7885, 78.299)
  line L104 (-48.7885, 78.299) -> (-48.7885, 83.299)
  line L105 (-48.7885, 83.299) -> (-53.1186, 85.799)
  line L106 (-42.9584, 85.799) -> (-47.2885, 83.299)
  line L107 (-47.2885, 83.299) -> (-47.2885, 78.299)
  line L108 (-47.2885, 78.299) -> (-42.9584, 75.799)
  line L109 (-42.9584, 75.799) -> (-38.6282, 78.299)
  line L110 (-38.6282, 78.299) -> (-38.6282, 83.299)
  line L111 (-38.6282, 83.299) -> (-42.9584, 85.799)
  line L112 (-32.7981, 85.799) -> (-37.1282, 83.299)
  line L113 (-37.1282, 83.299) -> (-37.1282, 78.299)
  line L114 (-37.1282, 78.299) -> (-32.7981, 75.799)
  line L115 (-32.7981, 75.799) -> (-28.468, 78.299)
  line L116 (-28.468, 78.299) -> (-28.468, 83.299)
  line L117 (-28.468, 83.299) -> (-32.7981, 85.799)
  line L118 (-22.6378, 85.799) -> (-26.968, 83.299)
  line L119 (-26.968, 83.299) -> (-26.968, 78.299)
  line L120 (-26.968, 78.299) -> (-22.6378, 75.799)
  line L121 (-22.6378, 75.799) -> (-18.3077, 78.299)
  line L122 (-18.3077, 78.299) -> (-18.3077, 83.299)
  line L123 (-18.3077, 83.299) -> (-22.6378, 85.799)
  line L124 (-12.4776, 85.799) -> (-16.8077, 83.299)
  line L125 (-16.8077, 83.299) -> (-16.8077, 78.299)
  line L126 (-16.8077, 78.299) -> (-12.4776, 75.799)
  line L127 (-12.4776, 75.799) -> (-8.1475, 78.299)
  line L128 (-8.1475, 78.299) -> (-8.1475, 83.299)
  line L129 (-8.1475, 83.299) -> (-12.4776, 85.799)
  line L130 (-109, 94.5981) -> (-113.3301, 92.0981)
  line L131 (-113.3301, 92.0981) -> (-113.3301, 87.0981)
  line L132 (-113.3301, 87.0981) -> (-109, 84.5981)
  line L133 (-109, 84.5981) -> (-104.6699, 87.0981)
  line L134 (-104.6699, 87.0981) -> (-104.6699, 92.0981)
  line L135 (-104.6699, 92.0981) -> (-109, 94.5981)
  line L136 (-98.8397, 94.5981) -> (-103.1699, 92.0981)
  line L137 (-103.1699, 92.0981) -> (-103.1699, 87.0981)
  line L138 (-103.1699, 87.0981) -> (-98.8397, 84.5981)
  line L139 (-98.8397, 84.5981) -> (-94.5096, 87.0981)
  line L140 (-94.5096, 87.0981) -> (-94.5096, 92.0981)
  line L141 (-94.5096, 92.0981) -> (-98.8397, 94.5981)
  line L142 (-88.6795, 94.5981) -> (-93.0096, 92.0981)
  line L143 (-93.0096, 92.0981) -> (-93.0096, 87.0981)
  line L144 (-93.0096, 87.0981) -> (-88.6795, 84.5981)
  line L145 (-88.6795, 84.5981) -> (-84.3494, 87.0981)
  line L146 (-84.3494, 87.0981) -> (-84.3494, 92.0981)
  line L147 (-84.3494, 92.0981) -> (-88.6795, 94.5981)
  line L148 (-78.5192, 94.5981) -> (-82.8494, 92.0981)
  line L149 (-82.8494, 92.0981) -> (-82.8494, 87.0981)
  line L150 (-82.8494, 87.0981) -> (-78.5192, 84.5981)
  line L151 (-78.5192, 84.5981) -> (-74.1891, 87.0981)
  line L152 (-74.1891, 87.0981) -> (-74.1891, 92.0981)
  line L153 (-74.1891, 92.0981) -> (-78.5192, 94.5981)
  line L154 (-68.359, 94.5981) -> (-72.6891, 92.0981)
  line L155 (-72.6891, 92.0981) -> (-72.6891, 87.0981)
  line L156 (-72.6891, 87.0981) -> (-68.359, 84.5981)
  line L157 (-68.359, 84.5981) -> (-64.0289, 87.0981)
  line L158 (-64.0289, 87.0981) -> (-64.0289, 92.0981)
  line L159 (-64.0289, 92.0981) -> (-68.359, 94.5981)
  line L160 (-58.1987, 94.5981) -> (-62.5289, 92.0981)
  line L161 (-62.5289, 92.0981) -> (-62.5289, 87.0981)
  line L162 (-62.5289, 87.0981) -> (-58.1987, 84.5981)
  line L163 (-58.1987, 84.5981) -> (-53.8686, 87.0981)
  line L164 (-53.8686, 87.0981) -> (-53.8686, 92.0981)
  line L165 (-53.8686, 92.0981) -> (-58.1987, 94.5981)
  line L166 (-48.0385, 94.5981) -> (-52.3686, 92.0981)
  line L167 (-52.3686, 92.0981) -> (-52.3686, 87.0981)
  line L168 (-52.3686, 87.0981) -> (-48.0385, 84.5981)
  line L169 (-48.0385, 84.5981) -> (-43.7084, 87.0981)
  line L170 (-43.7084, 87.0981) -> (-43.7084, 92.0981)
  line L171 (-43.7084, 92.0981) -> (-48.0385, 94.5981)
  line L172 (-37.8782, 94.5981) -> (-42.2084, 92.0981)
  line L173 (-42.2084, 92.0981) -> (-42.2084, 87.0981)
  line L174 (-42.2084, 87.0981) -> (-37.8782, 84.5981)
  line L175 (-37.8782, 84.5981) -> (-33.5481, 87.0981)
  line L176 (-33.5481, 87.0981) -> (-33.5481, 92.0981)
  line L177 (-33.5481, 92.0981) -> (-37.8782, 94.5981)
  line L178 (-27.718, 94.5981) -> (-32.0481, 92.0981)
  line L179 (-32.0481, 92.0981) -> (-32.0481, 87.0981)
  line L180 (-32.0481, 87.0981) -> (-27.718, 84.5981)
  line L181 (-27.718, 84.5981) -> (-23.3878, 87.0981)
  line L182 (-23.3878, 87.0981) -> (-23.3878, 92.0981)
  line L183 (-23.3878, 92.0981) -> (-27.718, 94.5981)
  line L184 (-17.5577, 94.5981) -> (-21.8878, 92.0981)
  line L185 (-21.8878, 92.0981) -> (-21.8878, 87.0981)
  line L186 (-21.8878, 87.0981) -> (-17.5577, 84.5981)
  line L187 (-17.5577, 84.5981) -> (-13.2276, 87.0981)
  line L188 (-13.2276, 87.0981) -> (-13.2276, 92.0981)
  line L189 (-13.2276, 92.0981) -> (-17.5577, 94.5981)
  line L190 (-7.3975, 94.5981) -> (-11.7276, 92.0981)
  line L191 (-11.7276, 92.0981) -> (-11.7276, 87.0981)
  line L192 (-11.7276, 87.0981) -> (-7.3975, 84.5981)
  line L193 (-7.3975, 84.5981) -> (-3.0673, 87.0981)
  line L194 (-3.0673, 87.0981) -> (-3.0673, 92.0981)
  line L195 (-3.0673, 92.0981) -> (-7.3975, 94.5981)
  line L196 (-103.9199, 103.3971) -> (-108.25, 100.8971)
  line L197 (-108.25, 100.8971) -> (-108.25, 95.8971)
  line L198 (-108.25, 95.8971) -> (-103.9199, 93.3971)
  line L199 (-103.9199, 93.3971) -> (-99.5897, 95.8971)
  line L200 (-99.5897, 95.8971) -> (-99.5897, 100.8971)
  line L201 (-99.5897, 100.8971) -> (-103.9199, 103.3971)
  line L202 (-93.7596, 103.3971) -> (-98.0897, 100.8971)
  line L203 (-98.0897, 100.8971) -> (-98.0897, 95.8971)
  line L204 (-98.0897, 95.8971) -> (-93.7596, 93.3971)
  line L205 (-93.7596, 93.3971) -> (-89.4295, 95.8971)
  line L206 (-89.4295, 95.8971) -> (-89.4295, 100.8971)
  line L207 (-89.4295, 100.8971) -> (-93.7596, 103.3971)
  line L208 (-83.5994, 103.3971) -> (-87.9295, 100.8971)
  line L209 (-87.9295, 100.8971) -> (-87.9295, 95.8971)
  line L210 (-87.9295, 95.8971) -> (-83.5994, 93.3971)
  line L211 (-83.5994, 93.3971) -> (-79.2692, 95.8971)
  line L212 (-79.2692, 95.8971) -> (-79.2692, 100.8971)
  line L213 (-79.2692, 100.8971) -> (-83.5994, 103.3971)
  line L214 (-73.4391, 103.3971) -> (-77.7692, 100.8971)
  line L215 (-77.7692, 100.8971) -> (-77.7692, 95.8971)
  line L216 (-77.7692, 95.8971) -> (-73.4391, 93.3971)
  line L217 (-73.4391, 93.3971) -> (-69.109, 95.8971)
  line L218 (-69.109, 95.8971) -> (-69.109, 100.8971)
  line L219 (-69.109, 100.8971) -> (-73.4391, 103.3971)
  line L220 (-63.2789, 103.3971) -> (-67.609, 100.8971)
  line L221 (-67.609, 100.8971) -> (-67.609, 95.8971)
  line L222 (-67.609, 95.8971) -> (-63.2789, 93.3971)
  line L223 (-63.2789, 93.3971) -> (-58.9487, 95.8971)
  line L224 (-58.9487, 95.8971) -> (-58.9487, 100.8971)
  line L225 (-58.9487, 100.8971) -> (-63.2789, 103.3971)
  line L226 (-53.1186, 103.3971) -> (-57.4487, 100.8971)
  line L227 (-57.4487, 100.8971) -> (-57.4487, 95.8971)
  line L228 (-57.4487, 95.8971) -> (-53.1186, 93.3971)
  line L229 (-53.1186, 93.3971) -> (-48.7885, 95.8971)
  line L230 (-48.7885, 95.8971) -> (-48.7885, 100.8971)
  line L231 (-48.7885, 100.8971) -> (-53.1186, 103.3971)
  line L232 (-42.9584, 103.3971) -> (-47.2885, 100.8971)
  line L233 (-47.2885, 100.8971) -> (-47.2885, 95.8971)
  line L234 (-47.2885, 95.8971) -> (-42.9584, 93.3971)
  line L235 (-42.9584, 93.3971) -> (-38.6282, 95.8971)
  line L236 (-38.6282, 95.8971) -> (-38.6282, 100.8971)
  line L237 (-38.6282, 100.8971) -> (-42.9584, 103.3971)
  line L238 (-32.7981, 103.3971) -> (-37.1282, 100.8971)
  line L239 (-37.1282, 100.8971) -> (-37.1282, 95.8971)
  line L240 (-37.1282, 95.8971) -> (-32.7981, 93.3971)
  line L241 (-32.7981, 93.3971) -> (-28.468, 95.8971)
  line L242 (-28.468, 95.8971) -> (-28.468, 100.8971)
  line L243 (-28.468, 100.8971) -> (-32.7981, 103.3971)
  line L244 (-22.6378, 103.3971) -> (-26.968, 100.8971)
  line L245 (-26.968, 100.8971) -> (-26.968, 95.8971)
  line L246 (-26.968, 95.8971) -> (-22.6378, 93.3971)
  line L247 (-22.6378, 93.3971) -> (-18.3077, 95.8971)
  line L248 (-18.3077, 95.8971) -> (-18.3077, 100.8971)
  line L249 (-18.3077, 100.8971) -> (-22.6378, 103.3971)
  line L250 (-12.4776, 103.3971) -> (-16.8077, 100.8971)
  line L251 (-16.8077, 100.8971) -> (-16.8077, 95.8971)
  line L252 (-16.8077, 95.8971) -> (-12.4776, 93.3971)
  line L253 (-12.4776, 93.3971) -> (-8.1475, 95.8971)
  line L254 (-8.1475, 95.8971) -> (-8.1475, 100.8971)
  line L255 (-8.1475, 100.8971) -> (-12.4776, 103.3971)
  line L256 (-109, 112.1962) -> (-113.3301, 109.6962)
  line L257 (-113.3301, 109.6962) -> (-113.3301, 104.6962)
  line L258 (-113.3301, 104.6962) -> (-109, 102.1962)
  line L259 (-109, 102.1962) -> (-104.6699, 104.6962)
  line L260 (-104.6699, 104.6962) -> (-104.6699, 109.6962)
  line L261 (-104.6699, 109.6962) -> (-109, 112.1962)
  line L262 (-98.8397, 112.1962) -> (-103.1699, 109.6962)
  line L263 (-103.1699, 109.6962) -> (-103.1699, 104.6962)
  line L264 (-103.1699, 104.6962) -> (-98.8397, 102.1962)
  line L265 (-98.8397, 102.1962) -> (-94.5096, 104.6962)
  line L266 (-94.5096, 104.6962) -> (-94.5096, 109.6962)
  line L267 (-94.5096, 109.6962) -> (-98.8397, 112.1962)
  line L268 (-88.6795, 112.1962) -> (-93.0096, 109.6962)
  line L269 (-93.0096, 109.6962) -> (-93.0096, 104.6962)
  line L270 (-93.0096, 104.6962) -> (-88.6795, 102.1962)
  line L271 (-88.6795, 102.1962) -> (-84.3494, 104.6962)
  line L272 (-84.3494, 104.6962) -> (-84.3494, 109.6962)
  line L273 (-84.3494, 109.6962) -> (-88.6795, 112.1962)
  line L274 (-78.5192, 112.1962) -> (-82.8494, 109.6962)
  line L275 (-82.8494, 109.6962) -> (-82.8494, 104.6962)
  line L276 (-82.8494, 104.6962) -> (-78.5192, 102.1962)
  line L277 (-78.5192, 102.1962) -> (-74.1891, 104.6962)
  line L278 (-74.1891, 104.6962) -> (-74.1891, 109.6962)
  line L279 (-74.1891, 109.6962) -> (-78.5192, 112.1962)
  line L280 (-68.359, 112.1962) -> (-72.6891, 109.6962)
  line L281 (-72.6891, 109.6962) -> (-72.6891, 104.6962)
  line L282 (-72.6891, 104.6962) -> (-68.359, 102.1962)
  line L283 (-68.359, 102.1962) -> (-64.0289, 104.6962)
  line L284 (-64.0289, 104.6962) -> (-64.0289, 109.6962)
  line L285 (-64.0289, 109.6962) -> (-68.359, 112.1962)
  line L286 (-58.1987, 112.1962) -> (-62.5289, 109.6962)
  line L287 (-62.5289, 109.6962) -> (-62.5289, 104.6962)
  line L288 (-62.5289, 104.6962) -> (-58.1987, 102.1962)
  line L289 (-58.1987, 102.1962) -> (-53.8686, 104.6962)
  line L290 (-53.8686, 104.6962) -> (-53.8686, 109.6962)
  line L291 (-53.8686, 109.6962) -> (-58.1987, 112.1962)
  line L292 (-48.0385, 112.1962) -> (-52.3686, 109.6962)
  line L293 (-52.3686, 109.6962) -> (-52.3686, 104.6962)
  line L294 (-52.3686, 104.6962) -> (-48.0385, 102.1962)
  line L295 (-48.0385, 102.1962) -> (-43.7084, 104.6962)
  line L296 (-43.7084, 104.6962) -> (-43.7084, 109.6962)
  line L297 (-43.7084, 109.6962) -> (-48.0385, 112.1962)
  line L298 (-37.8782, 112.1962) -> (-42.2084, 109.6962)
  line L299 (-42.2084, 109.6962) -> (-42.2084, 104.6962)
  line L300 (-42.2084, 104.6962) -> (-37.8782, 102.1962)
  line L301 (-37.8782, 102.1962) -> (-33.5481, 104.6962)
  line L302 (-33.5481, 104.6962) -> (-33.5481, 109.6962)
  line L303 (-33.5481, 109.6962) -> (-37.8782, 112.1962)
  line L304 (-27.718, 112.1962) -> (-32.0481, 109.6962)
  line L305 (-32.0481, 109.6962) -> (-32.0481, 104.6962)
  line L306 (-32.0481, 104.6962) -> (-27.718, 102.1962)
  line L307 (-27.718, 102.1962) -> (-23.3878, 104.6962)
  line L308 (-23.3878, 104.6962) -> (-23.3878, 109.6962)
  line L309 (-23.3878, 109.6962) -> (-27.718, 112.1962)
  line L310 (-17.5577, 112.1962) -> (-21.8878, 109.6962)
  line L311 (-21.8878, 109.6962) -> (-21.8878, 104.6962)
  line L312 (-21.8878, 104.6962) -> (-17.5577, 102.1962)
  line L313 (-17.5577, 102.1962) -> (-13.2276, 104.6962)
  line L314 (-13.2276, 104.6962) -> (-13.2276, 109.6962)
  line L315 (-13.2276, 109.6962) -> (-17.5577, 112.1962)
  line L316 (-7.3975, 112.1962) -> (-11.7276, 109.6962)
  line L317 (-11.7276, 109.6962) -> (-11.7276, 104.6962)
  line L318 (-11.7276, 104.6962) -> (-7.3975, 102.1962)
  line L319 (-7.3975, 102.1962) -> (-3.0673, 104.6962)
  line L320 (-3.0673, 104.6962) -> (-3.0673, 109.6962)
  line L321 (-3.0673, 109.6962) -> (-7.3975, 112.1962)
  line L322 (-103.9199, 120.9952) -> (-108.25, 118.4952)
  line L323 (-108.25, 118.4952) -> (-108.25, 113.4952)
  line L324 (-108.25, 113.4952) -> (-103.9199, 110.9952)
  line L325 (-103.9199, 110.9952) -> (-99.5897, 113.4952)
  line L326 (-99.5897, 113.4952) -> (-99.5897, 118.4952)
  line L327 (-99.5897, 118.4952) -> (-103.9199, 120.9952)
  line L328 (-93.7596, 120.9952) -> (-98.0897, 118.4952)
  line L329 (-98.0897, 118.4952) -> (-98.0897, 113.4952)
  line L330 (-98.0897, 113.4952) -> (-93.7596, 110.9952)
  line L331 (-93.7596, 110.9952) -> (-89.4295, 113.4952)
  line L332 (-89.4295, 113.4952) -> (-89.4295, 118.4952)
  line L333 (-89.4295, 118.4952) -> (-93.7596, 120.9952)
  line L334 (-83.5994, 120.9952) -> (-87.9295, 118.4952)
  line L335 (-87.9295, 118.4952) -> (-87.9295, 113.4952)
  line L336 (-87.9295, 113.4952) -> (-83.5994, 110.9952)
  line L337 (-83.5994, 110.9952) -> (-79.2692, 113.4952)
  line L338 (-79.2692, 113.4952) -> (-79.2692, 118.4952)
  line L339 (-79.2692, 118.4952) -> (-83.5994, 120.9952)
  line L340 (-73.4391, 120.9952) -> (-77.7692, 118.4952)
  line L341 (-77.7692, 118.4952) -> (-77.7692, 113.4952)
  line L342 (-77.7692, 113.4952) -> (-73.4391, 110.9952)
  line L343 (-73.4391, 110.9952) -> (-69.109, 113.4952)
  line L344 (-69.109, 113.4952) -> (-69.109, 118.4952)
  line L345 (-69.109, 118.4952) -> (-73.4391, 120.9952)
  line L346 (-63.2789, 120.9952) -> (-67.609, 118.4952)
  line L347 (-67.609, 118.4952) -> (-67.609, 113.4952)
  line L348 (-67.609, 113.4952) -> (-63.2789, 110.9952)
  line L349 (-63.2789, 110.9952) -> (-58.9487, 113.4952)
  line L350 (-58.9487, 113.4952) -> (-58.9487, 118.4952)
  line L351 (-58.9487, 118.4952) -> (-63.2789, 120.9952)
  line L352 (-53.1186, 120.9952) -> (-57.4487, 118.4952)
  line L353 (-57.4487, 118.4952) -> (-57.4487, 113.4952)
  line L354 (-57.4487, 113.4952) -> (-53.1186, 110.9952)
  line L355 (-53.1186, 110.9952) -> (-48.7885, 113.4952)
  line L356 (-48.7885, 113.4952) -> (-48.7885, 118.4952)
  line L357 (-48.7885, 118.4952) -> (-53.1186, 120.9952)
  line L358 (-42.9584, 120.9952) -> (-47.2885, 118.4952)
  line L359 (-47.2885, 118.4952) -> (-47.2885, 113.4952)
  line L360 (-47.2885, 113.4952) -> (-42.9584, 110.9952)
  line L361 (-42.9584, 110.9952) -> (-38.6282, 113.4952)
  line L362 (-38.6282, 113.4952) -> (-38.6282, 118.4952)
  line L363 (-38.6282, 118.4952) -> (-42.9584, 120.9952)
  line L364 (-32.7981, 120.9952) -> (-37.1282, 118.4952)
  line L365 (-37.1282, 118.4952) -> (-37.1282, 113.4952)
  line L366 (-37.1282, 113.4952) -> (-32.7981, 110.9952)
  line L367 (-32.7981, 110.9952) -> (-28.468, 113.4952)
  line L368 (-28.468, 113.4952) -> (-28.468, 118.4952)
  line L369 (-28.468, 118.4952) -> (-32.7981, 120.9952)
  line L370 (-22.6378, 120.9952) -> (-26.968, 118.4952)
  line L371 (-26.968, 118.4952) -> (-26.968, 113.4952)
  line L372 (-26.968, 113.4952) -> (-22.6378, 110.9952)
  line L373 (-22.6378, 110.9952) -> (-18.3077, 113.4952)
  line L374 (-18.3077, 113.4952) -> (-18.3077, 118.4952)
  line L375 (-18.3077, 118.4952) -> (-22.6378, 120.9952)
  line L376 (-12.4776, 120.9952) -> (-16.8077, 118.4952)
  line L377 (-16.8077, 118.4952) -> (-16.8077, 113.4952)
  line L378 (-16.8077, 113.4952) -> (-12.4776, 110.9952)
  line L379 (-12.4776, 110.9952) -> (-8.1475, 113.4952)
  line L380 (-8.1475, 113.4952) -> (-8.1475, 118.4952)
  line L381 (-8.1475, 118.4952) -> (-12.4776, 120.9952)
  line L382 (-109, 129.7942) -> (-113.3301, 127.2942)
  line L383 (-113.3301, 127.2942) -> (-113.3301, 122.2942)
  line L384 (-113.3301, 122.2942) -> (-109, 119.7942)
  line L385 (-109, 119.7942) -> (-104.6699, 122.2942)
  line L386 (-104.6699, 122.2942) -> (-104.6699, 127.2942)
  line L387 (-104.6699, 127.2942) -> (-109, 129.7942)
  line L388 (-98.8397, 129.7942) -> (-103.1699, 127.2942)
  line L389 (-103.1699, 127.2942) -> (-103.1699, 122.2942)
  line L390 (-103.1699, 122.2942) -> (-98.8397, 119.7942)
  line L391 (-98.8397, 119.7942) -> (-94.5096, 122.2942)
  line L392 (-94.5096, 122.2942) -> (-94.5096, 127.2942)
  line L393 (-94.5096, 127.2942) -> (-98.8397, 129.7942)
  line L394 (-88.6795, 129.7942) -> (-93.0096, 127.2942)
  line L395 (-93.0096, 127.2942) -> (-93.0096, 122.2942)
  line L396 (-93.0096, 122.2942) -> (-88.6795, 119.7942)
  line L397 (-88.6795, 119.7942) -> (-84.3494, 122.2942)
  line L398 (-84.3494, 122.2942) -> (-84.3494, 127.2942)
  line L399 (-84.3494, 127.2942) -> (-88.6795, 129.7942)
  line L400 (-78.5192, 129.7942) -> (-82.8494, 127.2942)
  line L401 (-82.8494, 127.2942) -> (-82.8494, 122.2942)
  line L402 (-82.8494, 122.2942) -> (-78.5192, 119.7942)
  line L403 (-78.5192, 119.7942) -> (-74.1891, 122.2942)
  line L404 (-74.1891, 122.2942) -> (-74.1891, 127.2942)
  line L405 (-74.1891, 127.2942) -> (-78.5192, 129.7942)
  line L406 (-68.359, 129.7942) -> (-72.6891, 127.2942)
  line L407 (-72.6891, 127.2942) -> (-72.6891, 122.2942)
  line L408 (-72.6891, 122.2942) -> (-68.359, 119.7942)
  line L409 (-68.359, 119.7942) -> (-64.0289, 122.2942)
  line L410 (-64.0289, 122.2942) -> (-64.0289, 127.2942)
  line L411 (-64.0289, 127.2942) -> (-68.359, 129.7942)
  line L412 (-58.1987, 129.7942) -> (-62.5289, 127.2942)
  line L413 (-62.5289, 127.2942) -> (-62.5289, 122.2942)
  line L414 (-62.5289, 122.2942) -> (-58.1987, 119.7942)
  line L415 (-58.1987, 119.7942) -> (-53.8686, 122.2942)
  line L416 (-53.8686, 122.2942) -> (-53.8686, 127.2942)
  line L417 (-53.8686, 127.2942) -> (-58.1987, 129.7942)
  line L418 (-48.0385, 129.7942) -> (-52.3686, 127.2942)
  line L419 (-52.3686, 127.2942) -> (-52.3686, 122.2942)
  line L420 (-52.3686, 122.2942) -> (-48.0385, 119.7942)
  line L421 (-48.0385, 119.7942) -> (-43.7084, 122.2942)
  line L422 (-43.7084, 122.2942) -> (-43.7084, 127.2942)
  line L423 (-43.7084, 127.2942) -> (-48.0385, 129.7942)
  line L424 (-37.8782, 129.7942) -> (-42.2084, 127.2942)
  line L425 (-42.2084, 127.2942) -> (-42.2084, 122.2942)
  line L426 (-42.2084, 122.2942) -> (-37.8782, 119.7942)
  line L427 (-37.8782, 119.7942) -> (-33.5481, 122.2942)
  line L428 (-33.5481, 122.2942) -> (-33.5481, 127.2942)
  line L429 (-33.5481, 127.2942) -> (-37.8782, 129.7942)
  line L430 (-27.718, 129.7942) -> (-32.0481, 127.2942)
  line L431 (-32.0481, 127.2942) -> (-32.0481, 122.2942)
  line L432 (-32.0481, 122.2942) -> (-27.718, 119.7942)
  line L433 (-27.718, 119.7942) -> (-23.3878, 122.2942)
  line L434 (-23.3878, 122.2942) -> (-23.3878, 127.2942)
  line L435 (-23.3878, 127.2942) -> (-27.718, 129.7942)
  line L436 (-17.5577, 129.7942) -> (-21.8878, 127.2942)
  line L437 (-21.8878, 127.2942) -> (-21.8878, 122.2942)
  line L438 (-21.8878, 122.2942) -> (-17.5577, 119.7942)
  line L439 (-17.5577, 119.7942) -> (-13.2276, 122.2942)
  line L440 (-13.2276, 122.2942) -> (-13.2276, 127.2942)
  line L441 (-13.2276, 127.2942) -> (-17.5577, 129.7942)
  line L442 (-7.3975, 129.7942) -> (-11.7276, 127.2942)
  line L443 (-11.7276, 127.2942) -> (-11.7276, 122.2942)